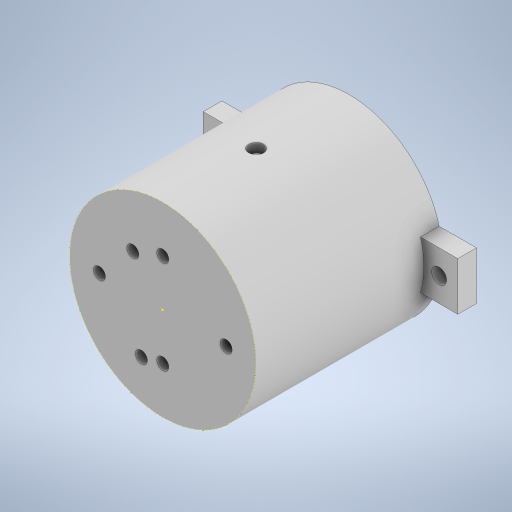
# Autodesk Inventor part: Hus_Til_Motor
Saved by Autodesk Inventor 2024 (Build 280153000, 153)
## iProperties
Created: 2024-03-01
Part Number: Hus_Til_Motor
Material: Generic
Document SubType Name: Modeling
Designer: jona3
Density: 1 g/cm^3
Appearance: Default
Author: jona3
Autodesk Inventor part; units mm, degrees
ref_plane "YZ Plane" through (0, 0, 0) normal (1, 0, 0) x (0, 1, 0)
ref_plane "XZ Plane" through (0, 0, 0) normal (0, 1, 0) x (-1, 0, 0)
ref_plane "XY Plane" through (0, 0, 0) normal (0, 0, 1) x (1, 0, 0)
sketch "Sketch1" plane through (0, 0, 0) normal (0, 0, 1) x (1, 0, 0)
  circle A0 centre (0, 0) radius 50
  dimension "d0" = 100
  constraints: 1 centre point, 1 coincident
  measures "d0" diameter of A0
extrude "Extrusion1" add sketch "Sketch1" along normal mid plane 100
sketch "Sketch2" plane through (0, 0, -50) normal (0, 0, -1) x (-1, 0, 0)
  circle A0 centre (0, 0) radius 45
  dimension "d3" = 90
  constraints: 1 centre point, 1 coincident
  measures "d3" diameter of A0
extrude "Extrusion2" cut sketch "Sketch2" against normal blind 95
sketch "Sketch5" plane through (0, 0, 50) normal (0, 0, 1) x (1, 0, 0)
  point P0 (0, 0)
sketch "Sketch7" plane through (0, 0, 50) normal (0, 0, 1) x (1, 0, 0)
  arc A0 (50, 0) -> (50, 0) centre (0, 0) ccw construction
  circle A1 centre (0, 0) radius 50 construction
sketch "Sketch8" plane through (0, 0, -50) normal (0, 0, -1) x (-1, 0, 0)
  arc A0 (48.2963, -12.941) -> (48.2963, 12.941) centre (0, 0) ccw
  line L0 (0, 0) -> (50, 0) construction
  line L1 (48.2963, 12.941) -> (68.2963, 12.941)
  line L2 (68.2963, 12.941) -> (68.2963, -12.941)
  line L3 (68.2963, -12.941) -> (48.2963, -12.941)
  line L4 (48.2963, 12.941) -> (-48.2963, 12.941) construction
  line L5 (48.2963, -12.941) -> (-48.2963, -12.941) construction
  circle A1 centre (0, 0) radius 50 construction
  arc A2 (-48.2963, 12.941) -> (-48.2963, -12.941) centre (0, 0) ccw
  line L6 (-48.2963, -12.941) -> (-68.2963, -12.941)
  line L7 (-68.2963, -12.941) -> (-68.2963, 12.941)
  line L8 (-68.2963, 12.941) -> (-48.2963, 12.941)
  dimension "d31" = 50
  dimension "d34" = 20
  dimension "d35" = 20
  constraints: 18 end point, 6 point on circle, 4 horizontal, 4 perpendicular, 2 centre point, 2 coincident
  measures "d31" radius of A0
  measures "d34" distance of L1.start L1.end
  measures "d35" distance of L5.end L6.end
extrude "Extrusion5" add sketch "Sketch8" against normal blind 10
sketch "Sketch9" plane through (0, 0, 50) normal (0, 0, 1) x (1, 0, 0)
  point P0 (0, 0)
sketch "Sketch10" plane through (0, 0, 50) normal (0, 0, 1) x (1, 0, 0)
  line L0 (-68.2963, -12.941) -> (-68.2963, 12.941) construction
  line L1 (-68.2963, -12.941) -> (-48.4721, 12.941) construction
  line L2 (-68.2963, 12.941) -> (-48.4721, -12.941) construction
  line L3 (48.2963, 12.941) -> (68.2963, 12.941) construction
  line L4 (48.2963, -12.941) -> (68.2963, 12.941) construction
  line L5 (68.2963, 12.941) -> (68.2963, -12.941) construction
  arc A0 (48.2963, -12.941) -> (48.2963, 12.941) centre (0, 0) ccw construction
  line L6 (68.2963, -12.941) -> (48.2963, 12.941) construction
  point P0 (-58.3842, 0)
  point P1 (58.2963, 0)
  constraints: 10 end point, 2 midpoint, 1 perpendicular
hole "Hole2" at (-58.3842, 0, 50) at (58.2963, 0, 50) direction (0, 0, -1) diameter 8 end through all counterbore diameter 11 counterbore depth 6.5
sketch "Sketch11" plane through (-68.2963, -12.941, -50) normal (0, -1, 0) x (1, 0, 0)
  line L0 (20, 0) -> (116.5926, 0) construction
  line L1 (118.2963, 100) -> (18.2963, 100) construction
  line L2 (20, 0) -> (118.2963, 100) construction
  line L3 (118.2963, 100) -> (18.2963, 100) construction
  line L4 (116.5926, 10) -> (116.5926, 0) construction
  line L5 (18.2963, 100) -> (116.5926, 0) construction
  point P0 (68.2963, 50)
  point P1 (68.2963, 50)
  constraints: 6 end point, 1 coincident, 1 collinear
hole "Hole3" at (0, -12.941, 0) direction (0, 1, 0) diameter 8 end through all
sketch "Sketch12" plane through (0, 0, 50) normal (0, 0, 1) x (1, 0, 0)
  circle A0 centre (0, 0) radius 42
  circle A1 centre (0, 0) radius 25
  line L0 (0, 70.0025) -> (0, -70.0004) projected
  line L1 (-95.6148, 0) -> (95.6148, 0) projected
  point P0 (0, 25)
  point P1 (0, -25)
  dimension "d52" = 84
  dimension "d53" = 50
  constraints: 2 centre point, 2 coincident, 2 point on circle, 2 point on line
  measures "d52" diameter of A0
  measures "d53" diameter of A1
hole "Hole4" at (0, 25, 50) at (0, -25, 50) direction (0, 0, -1) diameter 6.4 end through all
sketch "Sketch13" plane through (0, 0, 50) normal (0, 0, 1) x (1, 0, 0)
  circle A0 centre (0, 0) radius 34
  line L0 (0, 70.0025) -> (0, -70.0004) projected
  line L1 (-95.6148, 0) -> (95.6148, 0) projected
  point P0 (-34, 0)
  point P1 (34, 0)
  dimension "d61" = 68
  constraints: 2 point on circle, 2 point on line, 1 centre point, 1 coincident
  measures "d61" diameter of A0
hole "Hole5" at (-34, 0, 50) at (34, 0, 50) direction (0, 0, -1) diameter 6.4 end through all
sketch "Sketch14" plane through (0, 0, 50) normal (0, 0, 1) x (1, 0, 0)
  circle A0 centre (0, 0) radius 25
  line L0 (0, 0) -> (-11.4805, -27.7164)
  line L1 (0, 70.0025) -> (0, -70.0004) projected
  line L2 (-95.6148, 0) -> (95.6148, 0) projected
  dimension "d69" = 50
  dimension "d70" = 30
  constraints: 2 coincident, 2 end point, 1 centre point
  measures "d69" diameter of A0
  measures "d70" distance of L0.start L0.end
hole "Hole6" at (-11.4805, -27.7164, 50) direction (0, 0, -1) diameter 6.4 end through all
sketch "Sketch15" plane through (0, 0, 50) normal (0, 0, 1) x (1, 0, 0)
  circle A0 centre (0, 0) radius 25 construction
  line L0 (0, 0) -> (-16.0697, 19.1511) construction
  line L1 (0, 70.0025) -> (0, -70.0004) construction
  line L2 (-95.6148, 0) -> (95.6148, 0) construction
  dimension "d79" = 50
  dimension "d80" = 40
  constraints: 2 coincident, 2 end point, 3 other
  measures "d80" angle of L1 L0
hole "Hole7" at (-16.0697, 19.1511, 50) at (-16.0697, 19.1511, 50) direction (0, 0, -1) diameter 6.4 end through all
body "Solid1"
